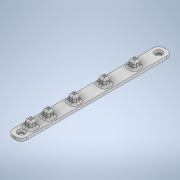
# Autodesk Inventor part: Piece 1
Saved by Autodesk Inventor 2022 (Build 260153000, 153)
## iProperties
Created: 2022-06-04
Part Number: Piece 1
Material: Générique
Document SubType Name: Modeling
Designer: timot
Density: 1 g/cm^3
Appearance: Par défaut
Author: timot
Autodesk Inventor part; units mm, degrees
ref_plane "YZ Plane" through (0, 0, 0) normal (1, 0, 0) x (0, 1, 0)
ref_plane "XZ Plane" through (0, 0, 0) normal (0, 1, 0) x (-1, 0, 0)
ref_plane "XY Plane" through (0, 0, 0) normal (0, 0, 1) x (1, 0, 0)
sketch "Esquisse1" plane through (0, 0, 0) normal (0, 1, 0) x (-1, 0, 0)
  line L0 (5, 45) -> (-5, 45)
  line L1 (-5, 45) -> (-5, -45)
  line L2 (-5, -45) -> (5, -45)
  line L3 (5, -45) -> (5, 45)
  line L4 (5, 45) -> (-5, -45) construction
  line L5 (-5, 45) -> (5, -45) construction
  line L6 (-5, 45) -> (5, 45)
  line L7 (5, 45) -> (5, 55)
  line L8 (5, 55) -> (-5, 55)
  line L9 (-5, 55) -> (-5, 45)
  line L10 (5, -45) -> (-5, -45)
  line L11 (-5, -45) -> (-5, -55)
  line L12 (-5, -55) -> (5, -55)
  line L13 (5, -55) -> (5, -45)
  point P0 (0, 0)
  dimension "d0" = 10
  dimension "d1" = 90
  dimension "d2" = 10
  dimension "d3" = 10
  constraints: 28 end point, 6 parallel, 3 horizontal, 3 perpendicular, 2 midpoint, 1 point on line
  measures "d0" distance of L2.end L1.end
  measures "d1" distance of L0.end L1.end
  measures "d2" distance of L7.end L6.end
  measures "d3" distance of L11.end L10.end
extrude "Extrusion1" add sketch "Esquisse1" along normal blind 2
sketch "Esquisse2" plane through (0, 2, 0) normal (0, 1, 0) x (1, 0, 0)
  line L0 (-5, 55) -> (-5, -55) projected
  line L1 (5, -55) -> (5, 55) projected
  line L2 (-5, -55) -> (5, -55)
  line L3 (5, -55) -> (5, -45)
  line L4 (5, -45) -> (-5, -45)
  line L5 (-5, -45) -> (-5, -55)
  line L6 (5, 55) -> (-5, 55) projected
  line L7 (-5, 55) -> (5, 55)
  line L8 (5, 55) -> (5, 45)
  line L9 (5, 45) -> (-5, 45)
  line L10 (-5, 45) -> (-5, 55)
  circle A0 centre (0, -50) radius 1.5
  circle A1 centre (0, 50) radius 1.5
  point P0 (0, 0)
  dimension "d6" = 10
  dimension "d7" = 10
  dimension "d8" = 3
  dimension "d9" = 3
  constraints: 16 end point, 4 parallel, 2 centre point, 2 horizontal, 2 perpendicular, 2 point on line
  measures "d6" distance of L3.end L2.end
  measures "d7" distance of L7.end L8.end
  measures "d8" diameter of A0
  measures "d9" diameter of A1
extrude "Extrusion2" cut sketch "Esquisse2" against normal blind 2 contours A0 | A1
chamfer "Chanfrein1" distance 1.25 angle 45 2 edges at (-1.5, 2, 50) (-1.5, 2, -50)
sketch "Esquisse3" plane through (0, 2, 0) normal (0, 1, 0) x (1, 0, 0)
  line L0 (-2.5, -45.6862) -> (2.5, -45.6862)
  line L1 (2.5, -45.6862) -> (2.5, -40.6862)
  line L2 (2.5, -40.6862) -> (-2.5, -40.6862)
  line L3 (-2.5, -40.6862) -> (-2.5, -45.6862)
  line L4 (-2.5, -45.6862) -> (2.5, -40.6862) construction
  line L5 (2.5, -45.6862) -> (-2.5, -40.6862) construction
  line L6 (-2.5, 29.855) -> (2.5, 29.855)
  line L7 (2.5, 29.855) -> (2.5, 34.855)
  line L8 (2.5, 34.855) -> (-2.5, 34.855)
  line L9 (-2.5, 34.855) -> (-2.5, 29.855)
  line L10 (-2.5, 29.855) -> (2.5, 34.855) construction
  line L11 (2.5, 29.855) -> (-2.5, 34.855) construction
  line L12 (-2.5, -32.8998) -> (2.5, -32.8998)
  line L13 (2.5, -32.8998) -> (2.5, -27.8998)
  line L14 (2.5, -27.8998) -> (-2.5, -27.8998)
  line L15 (-2.5, -27.8998) -> (-2.5, -32.8998)
  line L16 (-2.5, -32.8998) -> (2.5, -27.8998) construction
  line L17 (2.5, -32.8998) -> (-2.5, -27.8998) construction
  line L18 (-2.5, -13.9724) -> (2.5, -13.9724)
  line L19 (2.5, -13.9724) -> (2.5, -8.9724)
  line L20 (2.5, -8.9724) -> (-2.5, -8.9724)
  line L21 (-2.5, -8.9724) -> (-2.5, -13.9724)
  line L22 (-2.5, -13.9724) -> (2.5, -8.9724) construction
  line L23 (2.5, -13.9724) -> (-2.5, -8.9724) construction
  line L24 (-2.5, 7.9833) -> (2.5, 7.9833)
  line L25 (2.5, 7.9833) -> (2.5, 12.9833)
  line L26 (2.5, 12.9833) -> (-2.5, 12.9833)
  line L27 (-2.5, 12.9833) -> (-2.5, 7.9833)
  line L28 (-2.5, 7.9833) -> (2.5, 12.9833) construction
  line L29 (2.5, 7.9833) -> (-2.5, 12.9833) construction
  point P0 (0, 0)
  point P1 (0, -43.1862)
  point P2 (0, 32.355)
  point P3 (0, -30.3998)
  point P4 (0, -11.4724)
  point P5 (0, 10.4833)
  dimension "d15" = 5
  dimension "d16" = 5
  dimension "d17" = 5
  dimension "d18" = 5
  dimension "d19" = 5
  dimension "d20" = 5
  dimension "d21" = 5
  dimension "d22" = 5
  dimension "d23" = 5
  constraints: 60 end point, 10 midpoint, 10 parallel, 5 horizontal, 5 perpendicular
  measures "d15" distance of L2.end L1.end
  measures "d16" distance of L1.end L0.end
  measures "d17" distance of L8.end L7.end
  measures "d18" distance of L7.end L6.end
  measures "d19" distance of L14.end L13.end
  measures "d20" distance of L13.end L12.end
  measures "d21" distance of L20.end L19.end
  measures "d22" distance of L19.end L18.end
  measures "d23" distance of L25.end L24.end
extrude "Extrusion3" add sketch "Esquisse3" along normal blind 5
sketch "Esquisse4" plane through (0, 7, 0) normal (0, 1, 0) x (1, 0, 0)
  line L0 (-2.5, -40.6862) -> (-2.5, -45.6862) projected
  line L1 (2.5, -45.6862) -> (2.5, -40.6862) projected
  line L2 (-2.5, -45.6862) -> (2.5, -45.6862)
  line L3 (2.5, -45.6862) -> (2.5, -40.6862)
  line L4 (2.5, -40.6862) -> (-2.5, -40.6862)
  line L5 (-2.5, -40.6862) -> (-2.5, -45.6862)
  line L6 (-2.5, -32.8998) -> (-2.5, -27.8998) projected
  line L7 (2.5, -32.8998) -> (2.5, -27.8998) projected
  line L8 (-2.5, -32.8998) -> (2.5, -32.8998)
  line L9 (2.5, -32.8998) -> (2.5, -27.8998)
  line L10 (2.5, -27.8998) -> (-2.5, -27.8998)
  line L11 (-2.5, -27.8998) -> (-2.5, -32.8998)
  line L12 (-2.5, -8.9724) -> (-2.5, -13.9724) projected
  line L13 (2.5, -8.9724) -> (2.5, -13.9724) projected
  line L14 (-2.5, -13.9724) -> (2.5, -13.9724)
  line L15 (2.5, -13.9724) -> (2.5, -8.9724)
  line L16 (2.5, -8.9724) -> (-2.5, -8.9724)
  line L17 (-2.5, -8.9724) -> (-2.5, -13.9724)
  line L18 (-2.5, 7.9833) -> (-2.5, 12.9833) projected
  line L19 (2.5, 12.9833) -> (2.5, 7.9833) projected
  line L20 (-2.5, 7.9833) -> (2.5, 7.9833)
  line L21 (2.5, 7.9833) -> (2.5, 12.9833)
  line L22 (2.5, 12.9833) -> (-2.5, 12.9833)
  line L23 (-2.5, 12.9833) -> (-2.5, 7.9833)
  line L24 (-2.5, 29.855) -> (-2.5, 34.855) projected
  line L25 (2.5, 29.855) -> (2.5, 34.855) projected
  line L26 (-2.5, 29.855) -> (2.5, 29.855)
  line L27 (2.5, 29.855) -> (2.5, 34.855)
  line L28 (2.5, 34.855) -> (-2.5, 34.855)
  line L29 (-2.5, 34.855) -> (-2.5, 29.855)
  circle A0 centre (0, -43.1862) radius 1
  circle A1 centre (0, -30.3998) radius 1
  circle A2 centre (0, -11.4724) radius 1
  circle A3 centre (0, 10.4833) radius 1
  circle A4 centre (0, 32.355) radius 1
  point P0 (0, 0)
  dimension "d26" = 2
  dimension "d27" = 2
  constraints: 40 end point, 10 parallel, 5 centre point, 5 horizontal, 5 perpendicular
  measures "d26" diameter of A0
  measures "d27" diameter of A1
revolve "Révolution1" cut sketch "Esquisse4" angle 360 about axis through (2.5, 7, 45.6862) along (0, 0, -1) contours A0 | A1 | A2 | A3 | A4
fillet "Congé1" radius 1.5 60 edges at (2.5, 4.5, 45.6862) (2.5, 4.5, 40.6862) (2.5, 7, 43.1862) (0, 7, 45.6862) (-2.5, 7, 43.1862) (0, 7, 40.6862) (-2.5, 4.5, 45.6862) (-2.5, 4.5, 40.6862) (2.5, 2, 43.1862) (0, 2, 45.6862) (-2.5, 2, 43.1862) (0, 2, 40.6862) (-2.5, 4.5, 32.8998) (-2.5, 7, 30.3998) (-2.5, 4.5, 27.8998) (0, 7, 32.8998) (2.5, 7, 30.3998) (2.5, 4.5, 32.8998) (0, 2, 32.8998) (2.5, 2, 30.3998) (-2.5, 2, 30.3998) (0, 2, 27.8998) (0, 7, 13.9724) (2.5, 7, 11.4724) (0, 7, 8.9724) (-2.5, 7, 11.4724) (-2.5, 2, 11.4724) (-2.5, 4.5, 8.9724) (-2.5, 4.5, 13.9724) (0, 2, 8.9724) (2.5, 4.5, 8.9724) (2.5, 2, 11.4724) (0, 2, 13.9724) (2.5, 4.5, 13.9724) (0, 7, 27.8998) (2.5, 4.5, 27.8998) (0, 2, -7.9833) (2.5, 4.5, -7.9833) (0, 7, -7.9833) (2.5, 7, -10.4833) (0, 7, -12.9833) (-2.5, 7, -10.4833) (-2.5, 4.5, -7.9833) (2.5, 2, -10.4833) (2.5, 4.5, -12.9833) (-2.5, 2, -10.4833) (-2.5, 4.5, -12.9833) (0, 2, -12.9833) (0, 2, -29.855) (2.5, 2, -32.355) (2.5, 4.5, -29.855) (2.5, 4.5, -34.855) (2.5, 7, -32.355) (0, 7, -34.855) (-2.5, 7, -32.355) (0, 7, -29.855) (-2.5, 4.5, -29.855) (-2.5, 4.5, -34.855) (0, 2, -34.855) (-2.5, 2, -32.355)
fillet "Congé2" radius 4 4 edges at (5, 1, 55) (-5, 1, 55) (5, 1, -55) (-5, 1, -55)
